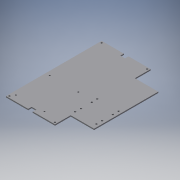
# Autodesk Inventor part: Part53
Saved by Autodesk Inventor 2016 (Build 200138000, 138)
## iProperties
Created: 2015-11-07
Part Number: Part53
Material: Generic
Document SubType Name: Modeling
Designer: Jufo
Density: 1 g/cm^3
Appearance: Default
Author: Jufo
Autodesk Inventor part; units mm, degrees
ref_plane "YZ Plane" through (0, 0, 0) normal (1, 0, 0) x (0, 1, 0)
ref_plane "XZ Plane" through (0, 0, 0) normal (0, 1, 0) x (-1, 0, 0)
ref_plane "XY Plane" through (0, 0, 0) normal (0, 0, 1) x (1, 0, 0)
sketch "Sketch1" plane through (0, 0, 0) normal (0, 1, 0) x (-1, 0, 0)
  line L0 (49.278, 4.7758) -> (49.278, -22.2242)
  line L1 (136.278, 144.7758) -> (136.278, -25.2242)
  line L2 (49.278, -22.2242) -> (87.278, -22.2242)
  line L3 (87.278, -22.2242) -> (87.278, -16.2242)
  line L4 (87.278, -16.2242) -> (95.278, -16.2242)
  line L5 (95.278, -16.2242) -> (95.278, -22.2242)
  line L6 (95.278, 141.7758) -> (95.278, 135.7758)
  line L7 (95.278, 135.7758) -> (87.278, 135.7758)
  line L8 (87.278, 135.7758) -> (87.278, 141.7758)
  line L9 (87.278, 141.7758) -> (49.278, 141.7758)
  line L10 (49.278, 141.7758) -> (49.278, 114.7758)
  line L11 (49.278, 4.7758) -> (9.278, 4.7758)
  line L12 (9.278, 4.7758) -> (9.278, 114.7758)
  line L13 (9.278, 114.7758) -> (49.278, 114.7758)
  line L14 (94.278, 136.7758) -> (94.278, 142.7758)
  line L15 (48.278, 142.7758) -> (134.278, 142.7758)
  line L16 (134.278, -23.2242) -> (48.278, -23.2242)
  line L17 (94.278, -23.2242) -> (94.278, -17.2242)
  line L18 (94.278, -17.2242) -> (88.278, -17.2242)
  line L19 (88.278, -17.2242) -> (88.278, -23.2242)
  line L20 (48.278, -23.2242) -> (48.278, 3.7758)
  line L21 (48.278, 3.7758) -> (24.278, 3.7758)
  line L22 (24.278, 115.7758) -> (48.278, 115.7758)
  line L23 (48.278, 115.7758) -> (48.278, 142.7758)
  line L24 (88.278, 142.7758) -> (88.278, 136.7758)
  line L25 (24.278, 3.7758) -> (8.278, 3.7758)
  line L26 (24.278, 115.7758) -> (8.278, 115.7758)
  line L27 (8.278, 115.7758) -> (8.278, 3.7758)
  line L28 (94.278, 136.7758) -> (88.278, 136.7758)
  line L29 (134.278, -23.2242) -> (134.278, 142.7758)
  line L30 (95.278, 141.7758) -> (134.278, 141.7758)
  line L31 (95.278, -22.2242) -> (134.278, -22.2242)
  line L32 (134.278, 141.7758) -> (133.278, 141.7758)
  line L33 (133.278, 141.7758) -> (133.278, -22.2242)
  line L34 (133.278, -22.2242) -> (134.278, -22.2242)
  line L35 (134.278, -22.2242) -> (134.278, 141.7758)
  point P0 (0, 0)
  point P1 (0, 0)
  dimension "d0" = 1
  dimension "d4" = 1
  dimension "d5" = 1
  dimension "d6" = 1
  dimension "d7" = 1
  dimension "d8" = 1
  dimension "d10" = 1
  dimension "d11" = 1
  dimension "d12" = 1
  dimension "d13" = 1
  dimension "d14" = 1
  dimension "d15" = 1
  dimension "d16" = 6
  dimension "d17" = 0
  dimension "d18" = 0
  dimension "d25" = 1
  constraints: 72 end point, 13 perpendicular, 5 point on line, 4 horizontal, 2 parallel
  measures "d0" distance from line of L6.start L14
  measures "d4" distance from line of L4.end L17
  measures "d5" distance between parallel lines of L4 L18
  measures "d6" distance between parallel lines of L19 L3
  measures "d7" distance between parallel lines of L20 L0
  measures "d8" distance between parallel lines of L11 L21
  measures "d10" distance between parallel lines of L16 L2
  measures "d11" distance from line of L22 L10.end
  measures "d12" distance between parallel lines of L10 L23
  measures "d13" distance between parallel lines of L24 L8
  measures "d14" distance between parallel lines of L15 L9
  measures "d15" distance between parallel lines of L7 L28
  measures "d16" distance of L24.start L24.end
  measures "d17" distance from line of L15 L14.end
  measures "d18" distance from line of L15 L24.start
  measures "d25" distance of L30.end L32.end
extrude "Extrusion2" add sketch "Sketch1" along normal blind 2 contours L11 L12 L13 L10 L9 L8 L7 L6 L30 L33 L31 L5 L4 L3 L2 L0
sketch "Sketch2" plane through (0, 2, 0) normal (0, 1, 0) x (1, 0, 0)
  circle A0 centre (-52.278, 19.2242) radius 1.5
  line L0 (-49.278, -4.7758) -> (-49.278, 22.2242) projected
  line L1 (-49.278, 22.2242) -> (-87.278, 22.2242) projected
  line L2 (-87.278, 16.2242) -> (-95.278, 16.2242) projected
  line L3 (-91.278, 16.2242) -> (-91.278, -30.1136)
  circle A1 centre (-130.278, 19.2242) radius 1.5
  line L4 (-9.278, -114.7758) -> (-9.278, -4.7758) projected
  line L5 (-9.278, -59.7758) -> (-80.3163, -59.7758)
  circle A2 centre (-52.278, -138.7758) radius 1.5
  circle A3 centre (-130.278, -138.7758) radius 1.5
  point P0 (0, 0)
  dimension "d26" = 3
  dimension "d27" = 3
  dimension "d28" = 3
  constraints: 4 centre point, 4 end point, 3 symmetric about line, 2 midpoint, 1 horizontal, 1 vertical, 3 other
  measures "d26" diameter of A0
  measures "d27" distance from line of A0.centre L0
  measures "d28" distance from line of L1 A0.centre
extrude "Extrusion3" cut sketch "Sketch2" against normal blind 10
sketch "Sketch3" plane through (0, 2, 0) normal (0, 1, 0) x (1, 0, 0)
  circle A0 centre (-77.278, -73.7758) radius 1.25
  circle A1 centre (-77.278, -73.7758) radius 1.25
  circle A2 centre (-77.278, -131.7758) radius 1.25
  circle A3 centre (-77.278, -131.7758) radius 1.25
  circle A4 centre (-126.278, -73.7758) radius 1.25
  circle A5 centre (-126.278, -73.7758) radius 1.25
  circle A6 centre (-126.278, -131.7758) radius 1.25
  circle A7 centre (-126.278, -131.7758) radius 1.25
  line L0 (-87.278, -141.7758) -> (-49.278, -141.7758) projected
  line L1 (-133.278, 22.2242) -> (-133.278, -141.7758) projected
  circle A8 centre (-77.278, -73.7758) radius 2.5
  circle A9 centre (-77.278, -131.7758) radius 2.5
  circle A10 centre (-126.278, -73.7758) radius 2.5
  circle A11 centre (-126.278, -131.7758) radius 2.5
  point P0 (0, 0)
  point P1 (40, -28)
  dimension "d31" = 49
  dimension "d32" = 58
  dimension "d33" = 49
  dimension "d34" = 58
  dimension "d35" = 10
  dimension "d36" = 10
  dimension "d37" = 7
  dimension "d38" = 7
  dimension "d70" = 5
  dimension "d71" = 5
  dimension "d72" = 5
  dimension "d73" = 5
  constraints: 12 centre point, 8 coincident
  measures "d31" distance of A5.centre A1.centre
  measures "d32" distance of A3.centre A1.centre
  measures "d33" distance of A7.centre A3.centre
  measures "d34" distance of A7.centre A5.centre
  measures "d35" distance from line of L0 A6.centre
  measures "d36" distance from line of L0 A3.centre
  measures "d37" distance from line of L1 A6.centre
  measures "d38" distance from line of L1 A4.centre
  measures "d70" diameter of A8
  measures "d71" diameter of A9
  measures "d72" diameter of A10
  measures "d73" diameter of A11
extrude "Extrusion4" add sketch "Sketch3" along normal blind 10
sketch "Sketch4" plane through (0, 0, 0) normal (0, -1, 0) x (1, 0, 0)
  circle A0 centre (-50.878, 67.7758) radius 1.5
  circle A1 centre (-50.878, 67.7758) radius 1.5
  circle A2 centre (-50.878, 105.7758) radius 1.5
  circle A3 centre (-50.878, 105.7758) radius 1.5
  circle A4 centre (-14.278, 67.7758) radius 1.5
  circle A5 centre (-14.278, 67.7758) radius 1.5
  circle A6 centre (-14.278, 105.7758) radius 1.5
  circle A7 centre (-14.278, 105.7758) radius 1.5
  line L0 (-9.278, 114.7758) -> (-9.278, 4.7758) projected
  line L1 (-49.278, 114.7758) -> (-9.278, 114.7758) projected
  point P0 (0, 0)
  point P1 (-48.9834, 91.5038)
  dimension "d53" = 38
  dimension "d54" = 36.6
  dimension "d55" = 38
  dimension "d56" = 36.6
  dimension "d57" = 38
  dimension "d58" = 38
  dimension "d59" = 5
  dimension "d60" = 9
  constraints: 8 centre point, 4 coincident
  measures "d53" distance of A5.centre A7.centre
  measures "d54" distance of A1.centre A5.centre
  measures "d55" distance of A3.centre A1.centre
  measures "d56" distance of A7.centre A3.centre
  measures "d57" vertical distance of A1.centre A7.centre
  measures "d58" vertical distance of A5.centre A3.centre
  measures "d59" distance from line of L0 A6.centre
  measures "d60" distance from line of L1 A6.centre
extrude "Extrusion5" cut sketch "Sketch4" against normal blind 10
sketch "Sketch5" plane through (0, 2, 0) normal (0, 1, 0) x (1, 0, 0)
  circle A0 centre (-50.478, -95.9758) radius 1.5
  circle A1 centre (-50.478, -95.9758) radius 1.5
  circle A2 centre (-50.478, -77.5758) radius 1.5
  circle A3 centre (-50.478, -77.5758) radius 1.5
  circle A4 centre (-14.278, -77.5758) radius 1.5
  circle A5 centre (-14.278, -77.5758) radius 1.5
  circle A6 centre (-14.278, -95.9758) radius 1.5
  circle A7 centre (-14.278, -95.9758) radius 1.5
  circle A8 centre (-14.278, -105.7758) radius 1.5 projected
  circle A9 centre (-14.278, -67.7758) radius 1.5 projected
  line L0 (-9.278, -114.7758) -> (-9.278, -4.7758) projected
  point P0 (0, 0)
  point P1 (0, 0)
  dimension "d43" = 18.4
  dimension "d44" = 36.2
  dimension "d45" = 18.4
  dimension "d46" = 36.2
  dimension "d47" = 36.2
  dimension "d48" = 36.2
  dimension "d49" = 9.8
  dimension "d50" = 9.8
  dimension "d51" = 5
  dimension "d52" = 5
  constraints: 8 centre point, 4 coincident
  measures "d43" distance of A7.centre A5.centre
  measures "d44" distance of A1.centre A7.centre
  measures "d45" distance of A1.centre A3.centre
  measures "d46" distance of A3.centre A5.centre
  measures "d47" horizontal distance of A5.centre A1.centre
  measures "d48" horizontal distance of A3.centre A7.centre
  measures "d49" distance of A8.centre A6.centre
  measures "d50" distance of A9.centre A4.centre
  measures "d51" distance from line of L0 A9.centre
  measures "d52" distance from line of L0 A4.centre
extrude "Extrusion6" cut sketch "Sketch5" against normal blind 10 contours A0 | A2 | A4 | A6
sketch "Sketch6" plane through (0, 2, 0) normal (0, 1, 0) x (1, 0, 0)
  line L0 (-133.278, 22.2242) -> (-133.278, -141.7758) projected
  line L1 (-133.278, 22.2242) -> (-133.278, 16.2242)
  line L2 (-133.278, 16.2242) -> (-130.278, 16.2242)
  line L3 (-130.278, 16.2242) -> (-130.278, 5.2242)
  line L4 (-130.278, 5.2242) -> (-133.278, 5.2242)
  line L5 (-133.278, 16.2242) -> (-133.278, 5.2242)
  line L6 (-133.278, -141.7758) -> (-133.278, -135.7758)
  line L7 (-133.278, -135.7758) -> (-130.278, -135.7758)
  line L8 (-130.278, -135.7758) -> (-130.278, -124.7758)
  line L9 (-130.278, -124.7758) -> (-133.278, -124.7758)
  line L10 (-133.278, -135.7758) -> (-133.278, -124.7758)
  point P0 (0, 0)
  dimension "d63" = 6
  dimension "d64" = 3
  dimension "d65" = 11
  dimension "d66" = 6
  dimension "d67" = 11
  constraints: 20 end point, 5 perpendicular, 4 point on line, 2 collinear, 1 vertical
  measures "d63" distance of L0.start L1.end
  measures "d64" distance of L1.end L2.end
  measures "d65" distance of L2.end L3.end
  measures "d66" distance of L0.end L6.end
  measures "d67" distance of L7.end L8.end
extrude "Extrusion7" cut sketch "Sketch6" against normal blind 10
equation "\"d36\" = d35"
equation "\"d38\" = d37"
body "Solid2"
